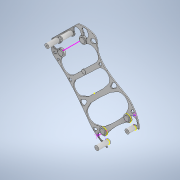
# Autodesk Inventor part: Schuh_Befestigung_alternative
Saved by Autodesk Inventor 2020.3 (Build 243373000, 373)
## iProperties
Created: 2020-03-04
Part Number: Schuh_Befestigung_alternative
Material: Generic
Document SubType Name: Modeling
Designer: Mara
Density: 1 g/cm^3
Appearance: Default
Mass: 24.396 g
Surface Area: 258.634 cm^2
Volume: 24.396 cm^3
d3: 5,563 mm
d8: 5,563 mm
d21: 60,427 mm
d22: 66,844 mm
d24: 47,207 mm
d29: 53,219 mm
d49: 6,361 mm
d51: 27,126 mm
d52: 44,927 mm
d53: 48,903 mm
d54: 29,968 mm
d55: 20,958 mm
d60: 67,034 mm
d61: 34,990 mm
d62: 27,853 mm
d63: 15,000 mm
d65: 20,850 mm
d71: 3,845 mm
d72: 5,442 mm
d73: 5,436 mm
d75: 5,541 mm
d76: 5,457 mm
d77: 3,113 mm
d78: 2,630 mm
d80: 3,207 mm
d82: 5,463 mm
d87: 1,600 mm
d88: 0,00 deg
d93: 1,000 mm
d94: 4,757 mm
d99: 1,000 mm
d100: 4,757 mm
d105: 17,100 mm
d106: 1,000 mm
d107: 0,00 deg
d108: 0,00 deg
d109: 4,757 mm
d110: 1,000 mm
d111: 11,100 mm
d112: 1,000 mm
d113: 0,00 deg
d114: 0,00 deg
d115: 2,049 mm
d117: 2,049 mm
d118: 3,300 mm
d119: 0,00 deg
d120: 2,049 mm
d121: 3,300 mm
d122: 0,00 deg
d123: 2,000 mm
d124: 0,00 deg
Author: Mara
Autodesk Inventor part; units mm, degrees
ref_plane "YZ Plane" through (0, 0, 0) normal (1, 0, 0) x (0, 1, 0)
ref_plane "XZ Plane" through (0, 0, 0) normal (0, 1, 0) x (-1, 0, 0)
ref_plane "XY Plane" through (0, 0, 0) normal (0, 0, 1) x (1, 0, 0)
sketch "Sketch1" plane through (0, 0, 0) normal (0, 0, 1) x (1, 0, 0)
  line L0 (-49.2977, 34.5359) -> (-47.8874, 33.1177) construction
  circle A0 centre (-52.4729, 29.968) radius 5.563
  circle A1 centre (-17.7815, 64.4351) radius 5.563
  circle A2 centre (14.4958, -44.9268) radius 5.563
  circle A3 centre (52.6405, -7.8239) radius 5.563
  circle A4 centre (-17.2221, 20.9576) radius 3.1804
  line L1 (-44.073, 65.9347) -> (-44.1303, 63.9354) construction
  line L2 (-59.1552, 49.3593) -> (-61.0015, 48.5894) construction
  line L3 (-42.1516, 65.9031) -> (-44.073, 65.9347) construction
  line L4 (-60.6997, 47.8234) -> (-61.0015, 48.5894) construction
  point P0 (0, 0)
  point P1 (-22.38, 61.3045)
  point P2 (-13.9364, 68.4553)
  point P3 (-12.7631, 66.8356)
  point P4 (-57.711, 28.0946)
  point P5 (-56.7093, 26.3625)
  point P6 (-49.5894, 25.2106)
  point P7 (10.1162, -41.4966)
  point P8 (9.143, -43.4122)
  point P9 (18.6755, -41.2556)
  point P10 (19.8991, -43.603)
  point P11 (47.2964, -9.3692)
  point P12 (58.0343, -9.1855)
  point P13 (55.8444, -3.2761)
  point P14 (-48.0932, 26.5378)
  point P15 (-14.6001, 59.8716)
  point P16 (48.0505, -4.6808)
  point P17 (-13.1915, 61.292)
  point P18 (49.4591, -3.2604)
  point P19 (49.4227, -12.3618)
  point P20 (19.1106, -41.8201)
  point P21 (48.0258, -10.9306)
  point P22 (17.7136, -40.3888)
  point P23 (11.2885, -49.4721)
  point P24 (9.8883, -48.0441)
  point P25 (57.2511, -4.7111)
  point P26 (55.8523, -3.2817)
  point P27 (-55.5021, 34.6339)
  point P28 (-53.6558, 35.4038)
  point P29 (-23.223, 65.5915)
  point P30 (-23.2803, 63.5921)
  point P31 (16.2732, -50.1982)
  point P32 (18.0227, -49.2289)
  point P33 (56.2951, -12.0181)
  point P34 (57.5423, -10.4544)
  point P35 (13.0651, -39.5509)
  point P36 (-16.7485, 17.8127)
  point P37 (-14.0533, 20.686)
  point P38 (47.9022, -4.9092)
  point P39 (47.1775, -6.7738)
  point P40 (-18.703, 58.9489)
  point P41 (-18.2564, 23.9652)
  point P42 (-16.7032, 58.9776)
  point P43 (-16.2565, 23.9879)
  point P44 (-47.4654, 27.5447)
  point P45 (-20.389, 20.6653)
  point P46 (-46.932, 29.4728)
  point P47 (-19.9371, 22.614)
  dimension "d3" = 5.563
  dimension "d8" = 5.563
  dimension "d21" = 60.4275
  dimension "d22" = 66.8436
  dimension "d24" = 47.2075
  dimension "d29" = 53.2188
  dimension "d49" = 6.3609
  dimension "d51" = 27.126
  dimension "d52" = 44.9268
  dimension "d53" = 48.9027
  dimension "d54" = 29.968
  dimension "d55" = 20.9576
  dimension "d60" = 67.0343
  dimension "d61" = 34.9897
  dimension "d62" = 27.8525
  dimension "d63" = 15
  dimension "d65" = 20.85
  dimension "d71" = 3.8451
  dimension "d72" = 5.4415
  dimension "d73" = 5.4358
  dimension "d75" = 5.5409
  dimension "d76" = 5.4575
  dimension "d77" = 3.1128
  dimension "d78" = 2.6305
  dimension "d80" = 3.2073
  dimension "d82" = 5.463
  dimension "d145" = 53.2132
  constraints: 10 end point, 6 point on circle, 1 centre point, 50 other
  measures "d3" distance of L0.start point (-52.473, 29.968)
  measures "d8" distance of point (-22.38, 61.305) point (-17.782, 64.435)
  measures "d21" distance of point (-52.473, 29.968) point (0, 0)
  measures "d22" distance of point (0, 0) point (-17.782, 64.435)
  measures "d24" distance of point (0, 0) point (14.496, -44.927)
  measures "d29" distance of point (0, 0) point (52.641, -7.824)
  measures "d49" diameter of A4
  measures "d51" distance of point (0, 0) A4.centre
  measures "d52" vertical distance of point (0, 0) point (14.496, -44.927)
  measures "d53" distance of point (-52.473, 29.968) point (-17.782, 64.435)
  measures "d54" vertical distance of point (0, 0) point (-52.473, 29.968)
  measures "d55" vertical distance of A4.centre point (0, 0)
  measures "d60" distance of A4.end point (47.902, -4.909)
  measures "d61" vertical distance of point (-16.703, 58.978) point (-16.256, 23.988)
  measures "d62" distance of point (-46.932, 29.473) point (-19.937, 22.614)
  measures "d63" distance of point (-53.656, 35.404) L2.start
  measures "d65" horizontal distance of point (-23.28, 63.592) L1.end
  measures "d71" horizontal distance of point (-13.936, 68.455) point (-17.782, 64.435)
  measures "d72" horizontal distance of point (-17.782, 64.435) point (-23.223, 65.591)
  measures "d73" vertical distance of point (-52.473, 29.968) point (-53.656, 35.404)
  measures "d75" horizontal distance of point (-52.473, 29.968) point (-46.932, 29.473)
  measures "d76" vertical distance of point (-17.782, 64.435) point (-16.703, 58.978)
  measures "d77" vertical distance of point (52.641, -7.824) point (57.251, -4.711)
  measures "d78" vertical distance of point (52.641, -7.824) point (57.542, -10.454)
  measures "d80" horizontal distance of point (14.496, -44.927) point (11.289, -49.472)
  measures "d82" horizontal distance of point (52.641, -7.824) point (47.178, -6.774)
  measures "d145" distance of point (52.641, -7.824) point (14.496, -44.927)
extrude "Extrusion3" add sketch "Sketch1" against normal blind 1.6
sketch "Sketch3" plane through (0, 0, 0) normal (0, 0, 1) x (1, 0, 0)
  circle A0 centre (20.7546, -56.5669) radius 2.3783
  circle A1 centre (20.7546, -56.5669) radius 3.3783
  circle A2 centre (-58.3828, 44.2123) radius 2.3783
  circle A3 centre (-58.3828, 44.2123) radius 3.3783
  circle A4 centre (52.6405, -7.8239) radius 5.563 projected
  circle A5 centre (14.4958, -44.9268) radius 5.563 projected
  point P0 (0, 0)
  point P1 (49.4227, -12.3618)
  point P2 (57.2511, -4.7111)
  point P3 (11.2885, -49.4721)
  point P4 (19.1106, -41.8201)
  dimension "d93" = 1
  dimension "d94" = 4.7566
  dimension "d99" = 1
  dimension "d100" = 4.7566
  constraints: 4 centre point, 2 coincident
  measures "d93" radial gap between concentric circles of A1 A0
  measures "d94" diameter of A0
  measures "d99" radial gap between concentric circles of A3 A2
  measures "d100" diameter of A2
extrude "Extrusion5" add sketch "Sketch3" along normal blind 17.1 and the other way blind 1 contours A1 | A3
sketch "Sketch6" plane through (0, 0, 0) normal (0, 0, 1) x (1, 0, 0)
  circle A0 centre (62.8402, -15.6905) radius 2.3785
  circle A1 centre (62.8402, -15.6905) radius 3.3785
  point P0 (0, 0)
  dimension "d109" = 4.757
  dimension "d110" = 1
  constraints: 2 centre point, 1 coincident
  measures "d109" diameter of A0
  measures "d110" radial gap between concentric circles of A1 A0
extrude "Extrusion6" add sketch "Sketch6" along normal blind 11.1 and the other way blind 1
sketch "Sketch7" plane through (-58.3828, 44.2123, 17.1) normal (0, 0, 1) x (1, 0, 0)
  circle A0 centre (0, 0) radius 3.3783
  circle A1 centre (0, 0) radius 3.3783 projected
  circle A2 centre (0, 0) radius 1.3297
  circle A3 centre (79.1375, -100.7793) radius 3.3783
  circle A4 centre (79.1375, -100.7793) radius 3.3783 projected
  circle A5 centre (79.1375, -100.7793) radius 1.3293
  point P0 (58.3828, -44.2123)
  dimension "d115" = 2.0486
  dimension "d117" = 2.049
  constraints: 4 centre point, 4 coincident, 2 concentric
  measures "d115" radial gap between concentric circles of A0 A2
  measures "d117" radial gap between concentric circles of A3 A5
extrude "Extrusion7" add sketch "Sketch7" against normal blind 3.3
sketch "Sketch8" plane through (62.8402, -15.6905, 11.1) normal (0, 0, 1) x (1, 0, 0)
  circle A0 centre (0, 0) radius 3.3785
  circle A1 centre (0, 0) radius 3.3785 projected
  circle A2 centre (0, 0) radius 1.3295
  point P0 (-62.8402, 15.6905)
  dimension "d120" = 2.049
  constraints: 2 centre point, 2 coincident, 1 concentric
  measures "d120" radial gap between concentric circles of A0 A2
extrude "Extrusion8" add sketch "Sketch8" against normal blind 3.3
sketch "Sketch9" plane through (0, 0, -1.6) normal (0, 0, -1) x (-1, 0, 0)
  circle A0 centre (58.3828, 44.2123) radius 2.3783
  circle A1 centre (58.3828, 44.2123) radius 2.3783 projected
  circle A2 centre (36.8834, 64.7402) radius 2.3783
  arc A3 (34.5051, 64.7402) -> (34.5051, 64.7402) centre (36.8834, 64.7402) ccw projected
  point P0 (0, 0)
  point P1 (56.0045, 44.2123)
  point P2 (56.0045, 44.2123)
  constraints: 2 centre point, 2 coincident, 2 concentric
extrude "Extrusion9" cut sketch "Sketch9" against normal blind 2
sketch "Sketch10" plane through (0, 0, 0) normal (0, 0, 1) x (1, 0, 0)
  circle A0 centre (52.6405, -7.8239) radius 5.563 projected
  circle A1 centre (62.8402, -15.6905) radius 3.3785 projected
  circle A2 centre (14.4958, -44.9268) radius 5.563 projected
  circle A3 centre (20.7546, -56.5669) radius 3.3783 projected
  circle A4 centre (20.7546, -56.5669) radius 3.3783 projected
  circle A5 centre (14.4958, -44.9268) radius 5.563 projected
  circle A6 centre (20.7546, -56.5669) radius 1.3293 projected
  line L0 (3.9093, -56.6581) -> (11.2885, -49.4721) projected
  circle A7 centre (62.8402, -15.6905) radius 1.3295 projected
  circle A8 centre (62.8402, -15.6905) radius 1.3295 projected
  circle A9 centre (-36.8834, 64.7402) radius 1.3293
  circle A10 centre (-36.8834, 64.7402) radius 2.3783 projected
  circle A11 centre (-58.3828, 44.2123) radius 2.3783 projected
  line L1 (-49.2977, 34.5359) -> (-22.38, 61.3045) projected
  point P0 (0, 0)
  point P1 (49.4227, -12.3618)
  point P2 (16.2829, -50.1949)
  point P3 (19.1106, -41.8201)
  point P4 (18.3621, -54.1818)
  point P5 (5.9631, -54.6581)
  point P6 (65.1179, 2.9774)
  point P7 (63.0109, 0.9182)
  point P8 (62.3382, -12.3495)
  point P9 (-57.2083, 46.2804)
  point P10 (-39.1976, 64.1914)
  point P11 (-56.04, 44.6216)
  point P12 (-37.948, 62.6134)
  constraints: 5 point on circle, 1 centre point, 1 point on line, 6 other
sketch "Sketch11" plane through (0, 0, 0) normal (0, 0, 1) x (1, 0, 0)
  circle A0 centre (-52.4729, 29.968) radius 5.563
  circle A1 centre (-52.4729, 29.968) radius 5.563 projected
  circle A2 centre (-52.4729, 29.968) radius 5.563 projected
  circle A3 centre (-52.4729, 29.968) radius 5.563 projected
  circle A4 centre (-17.7815, 64.4351) radius 5.563
  circle A5 centre (14.4958, -44.9268) radius 5.563
  circle A6 centre (52.6405, -7.8239) radius 5.563
  circle A7 centre (52.6405, -7.8239) radius 5.563 projected
  point P0 (0, 0)
  point P1 (-49.2977, 34.5359)
  point P2 (-53.6558, 35.4038)
  point P3 (-56.7093, 26.3625)
  point P4 (-49.5894, 25.2106)
  point P5 (-55.5021, 34.6339)
  point P6 (-57.711, 28.0946)
  point P7 (-13.9364, 68.4553)
  point P8 (-12.2185, 64.4351)
  point P9 (-23.223, 65.5915)
  point P10 (20.0588, -44.9268)
  point P11 (11.2885, -49.4721)
  point P12 (10.1162, -41.4966)
  point P13 (55.8523, -3.2817)
  point P14 (58.2035, -7.8239)
  point P15 (58.2035, -7.8239)
  constraints: 11 point on circle, 4 centre point, 4 concentric
extrude "Extrusion11" add sketch "Sketch11" along normal blind 0.8
sketch "Sketch12" plane through (-52.4729, 29.968, 0.8) normal (0, 0, 1) x (1, 0, 0)
  circle A0 centre (0, 0) radius 3.9985
  circle A1 centre (0, 0) radius 5.563 projected
  circle A2 centre (34.6914, 34.4671) radius 5.563 projected
  circle A3 centre (34.6914, 34.4671) radius 3.9985
  circle A4 centre (66.9687, -74.8947) radius 5.563 projected
  circle A5 centre (66.9687, -74.8947) radius 3.9985
  circle A6 centre (105.1134, -37.7919) radius 5.563 projected
  circle A7 centre (105.1134, -37.7919) radius 3.9985
  point P0 (52.4729, -29.968)
  dimension "d138" = 7.997
  dimension "d139" = 1.5645
  dimension "d140" = 7.997
  dimension "d141" = 7.997
  dimension "d142" = 7.997
  constraints: 4 centre point, 3 coincident
  measures "d138" diameter of A0
  measures "d139" radial gap between concentric circles of A0 A1
  measures "d140" diameter of A3
  measures "d141" diameter of A5
  measures "d142" diameter of A7
extrude "Extrusion12" add sketch "Sketch12" along normal blind 1 contours A0 | A3 | A5 | A7
sketch "Sketch13" plane through (-52.4729, 29.968, -1.6) normal (0, 0, -1) x (-1, 0, 0)
  arc A0 (-72.037, -95.4941) -> (-57.5443, -87.63) centre (-91.5548, -42.2379) ccw
  arc A1 (-57.5443, -87.63) -> (-44.0595, -74.0172) centre (-90.3784, -41.6193) ccw
  arc A2 (-20.5029, -42.7299) -> (-44.0595, -74.0172) centre (333.3705, -333.6762) ccw
  arc A3 (11.5166, -11.7542) -> (-20.5029, -42.7299) centre (138.9353, -175.5039) ccw
  arc A4 (16.0716, -3.8932) -> (15.4549, 11.4349) centre (-36.7536, 1.658) ccw
  arc A5 (11.5166, -11.7542) -> (16.0716, -3.8932) centre (2.1813, -1.0948) ccw
  line L0 (-25.7779, 51.9966) -> (15.4549, 11.4349)
  arc A6 (-25.7779, 51.9966) -> (-48.9728, 50.6804) centre (-34.8172, 6.2592) ccw
  arc A7 (-48.9728, 50.6804) -> (-54.7622, 45.0409) centre (-46.23, 42.0732) ccw
  arc A8 (-54.7622, 45.0409) -> (-56.0589, 39.2709) centre (-33.7926, 37.2978) ccw
  arc A9 (-56.5711, 33.7036) -> (-56.0589, 39.2709) centre (-281.8966, 57.2432) ccw
  arc A10 (-61.9243, 20.4575) -> (-56.5711, 33.7036) centre (-82.7996, 36.5985) ccw
  arc A11 (-72.0738, 10.1778) -> (-61.9243, 20.4575) centre (-99.4976, 47.4048) ccw
  arc A12 (-85.6338, 0.7644) -> (-72.0738, 10.1778) centre (-156.7554, 117.6883) ccw
  arc A13 (-103.5397, -9.3778) -> (-85.6338, 0.7644) centre (-553.714, 806.2763) ccw
  arc A14 (-103.5397, -9.3778) -> (-111.1126, -16.6996) centre (-85.4929, -35.6208) ccw
  arc A15 (-111.1126, -16.6996) -> (-120.4873, -33.6887) centre (-70.9711, -49.9311) ccw
  arc A16 (-120.4873, -33.6887) -> (-122.6827, -44.6984) centre (-77.4176, -48.0005) ccw
  line L1 (-122.6827, -44.6984) -> (-72.037, -95.4941)
  point P0 (-52.4729, -29.968)
  point P1 (-52.4749, -29.9699)
  constraints: 34 point on circle, 17 centre point, 4 end point
extrude "Extrusion13" add sketch "Sketch13" against normal blind 1.4
sketch "Sketch14" plane through (-52.4729, 29.968, -0.2) normal (0, 0, 1) x (1, 0, 0)
  arc A0 (30.7294, 38.3722) -> (19.1761, 37.6395) centre (24.7883, 40.598) ccw
  circle A1 centre (34.6914, 34.4671) radius 5.563 projected
  circle A2 centre (0, 0) radius 5.563 projected
  arc A3 (12.7593, 31.1185) -> (19.1761, 37.6395) centre (15.6189, 34.7222) ccw
  arc A4 (-8.6985, 10.4856) -> (-1.7496, 16.8027) centre (-5.8638, 14.3479) ccw
  arc A5 (-8.6985, 10.4856) -> (-14.5663, 7.4416) centre (-10.1859, 6.1752) ccw
  arc A6 (-14.5663, 7.4416) -> (-9.8157, 0) centre (-9.8062, 5.2432) ccw
  line L0 (-9.8157, 0) -> (-5.563, 0)
  arc A7 (12.7593, 31.1185) -> (-1.7496, 16.8027) centre (15.095, 14.2412) ccw
  arc A8 (38.6534, 38.3722) -> (41.5234, 48.802) centre (35.6734, 44.802) ccw
  arc A9 (41.5234, 48.802) -> (32.4139, 48.802) centre (36.9687, 47.054) ccw
  arc A10 (32.4139, 48.802) -> (34.3546, 44.168) centre (38.985, 48.8306) ccw
  arc A11 (34.6914, 40.0301) -> (34.3546, 44.168) centre (30.0196, 41.7326) ccw
  arc A12 (-10.4024, -4.3192) -> (-10.7489, -7.2712) centre (-11.1698, -5.7254) ccw
  line L1 (-10.4024, -4.3192) -> (-8.7851, -5.1021)
  line L2 (-8.7851, -5.1021) -> (-8.0664, -6.3471)
  line L3 (-8.0664, -6.3471) -> (-10.7489, -7.2712)
  arc A13 (52.4729, 37.6395) -> (49.4895, 44.168) centre (51.2863, 41.0432) ccw
  line L4 (49.4895, 44.168) -> (46.4093, 41.7326)
  line L5 (46.4093, 41.7326) -> (45.7933, 38.3722)
  line L6 (45.7933, 38.3722) -> (49.4895, 37.0246)
  line L7 (49.4895, 37.0246) -> (52.4729, 37.6395)
  arc A14 (30.7294, 38.3722) -> (38.985, 30.9299) centre (34.6914, 34.4671) ccw
  arc A15 (55.1671, 13.4743) -> (38.985, 30.9299) centre (46.4011, 21.5764) ccw
  arc A16 (1.28, -5.342) -> (19.8493, -21.2046) centre (10.9401, -12.8338) ccw
  line L8 (55.1671, 13.4743) -> (35.2508, -5.8299)
  circle A17 centre (35.2508, -9.0103) radius 3.1804 projected
  line L9 (19.8493, -21.2046) -> (32.0878, -9.3423)
  arc A18 (35.2508, -5.8299) -> (32.0878, -9.3423) centre (35.2508, -9.0103) ccw
  arc A19 (-6.871, -11.994) -> (-4.2674, -13.6642) centre (-5.4464, -12.6376) ccw
  line L10 (-4.2674, -13.6642) -> (-3.5379, -11.6631)
  line L11 (-3.5379, -11.6631) -> (-3.5379, -10.1027)
  line L12 (-3.5379, -10.1027) -> (-5.2195, -10.6821)
  line L13 (-5.2195, -10.6821) -> (-6.871, -11.994)
  arc A20 (12.2359, -29.3287) -> (15.4882, -32.0996) centre (13.862, -30.7141) ccw
  line L14 (15.4882, -32.0996) -> (16.4068, -31.287)
  line L15 (16.4068, -31.287) -> (16.5087, -29.968)
  line L16 (16.5087, -29.968) -> (15.9257, -28.4554)
  line L17 (15.9257, -28.4554) -> (13.1141, -28.5518)
  line L18 (13.1141, -28.5518) -> (12.2359, -29.3287)
  line L19 (59.4941, 15.0713) -> (60.3209, 15.9025)
  line L20 (59.2335, 12.27) -> (59.4941, 15.0713)
  line L21 (60.7094, 11.5997) -> (59.2335, 12.27)
  arc A21 (62.8971, 12.4938) -> (60.3209, 15.9025) centre (61.609, 14.1982) ccw
  line L22 (62.0321, 11.6243) -> (60.7094, 11.5997)
  line L23 (62.8971, 12.4938) -> (62.0321, 11.6243)
  arc A22 (30.7294, -54.7515) -> (37.277, -53.8855) centre (33.6979, -52.0102) ccw
  arc A23 (30.9665, -49.4464) -> (30.7294, -54.7515) centre (35.9638, -52.3276) ccw
  line L24 (37.277, -53.8855) -> (40.5855, -48.023)
  line L25 (30.9665, -49.4464) -> (38.4312, -45.8872)
  line L26 (38.4312, -45.8872) -> (40.2815, -47.1403)
  line L27 (40.2815, -47.1403) -> (40.5855, -48.023)
  arc A24 (86.5361, -0.0477) -> (81.2358, -0.3747) centre (84.2014, -5.3224) ccw
  line L28 (77.8037, -7.8987) -> (79.0881, -9.7275)
  line L29 (81.2358, -0.3747) -> (77.8037, -7.8987)
  line L30 (79.0881, -9.7275) -> (79.9758, -10.0165)
  arc A25 (85.7813, -6.609) -> (86.5361, -0.0477) centre (83.8456, -3.0622) ccw
  line L31 (85.7813, -6.609) -> (79.9758, -10.0165)
  arc A26 (73.8906, -7.0676) -> (58.0057, 6.9803) centre (65.8511, -0.1534) ccw
  arc A27 (20.6597, -29.968) -> (34.6989, -43.3595) centre (28.9526, -35.3288) ccw
  line L32 (58.0057, 6.9803) -> (21.3156, -27.7089)
  line L33 (21.3156, -27.7089) -> (20.6597, -29.968)
  line L34 (73.8906, -7.0676) -> (66.1837, -17.0703)
  line L35 (66.1837, -17.0703) -> (42.5062, -39.8702)
  line L36 (42.5062, -39.8702) -> (34.6989, -43.3595)
  arc A28 (105.6225, -25.3812) -> (86.5361, -11.0203) centre (93.8695, -21.1376) ccw
  line L37 (105.6225, -25.3812) -> (102.2106, -33.0462)
  circle A29 centre (105.1134, -37.7919) radius 5.563 projected
  line L38 (86.5361, -11.0203) -> (76.6806, -17.0499)
  line L39 (76.6806, -17.0499) -> (58.7599, -33.6007)
  line L40 (58.7599, -33.6007) -> (45.7408, -47.2708)
  line L41 (45.7408, -47.2708) -> (42.5558, -54.0083)
  arc A30 (42.5558, -54.0083) -> (56.8453, -71.9544) centre (51.9326, -61.2041) ccw
  line L42 (56.8453, -71.9544) -> (62.9636, -71.0339)
  arc A31 (38.6534, 38.3722) -> (34.6914, 40.0301) centre (34.6914, 34.4671) ccw
  arc A32 (114.4913, -25.8116) -> (111.2892, -23.4614) centre (113.0557, -24.4111) ccw
  line L43 (111.2892, -23.4614) -> (110.1208, -25.8116)
  line L44 (114.4913, -25.8116) -> (113.4337, -27.1923)
  line L45 (113.4337, -27.1923) -> (110.9367, -27.9267)
  line L46 (110.9367, -27.9267) -> (110.1208, -25.8116)
  arc A33 (50.8398, -77.9602) -> (53.4319, -81.7313) centre (52.6095, -79.5202) ccw
  line L47 (50.8398, -77.9602) -> (51.9326, -77.0845)
  line L48 (51.9326, -77.0845) -> (55.1671, -76.6058)
  line L49 (55.1671, -76.6058) -> (56.7359, -77.1778)
  arc A34 (53.4319, -81.7313) -> (56.7359, -77.1778) centre (51.0863, -76.5539) ccw
  arc A35 (119.1392, -33.3562) -> (108.6217, -33.4746) centre (113.9354, -38.3015) ccw
  circle A36 centre (115.3131, -45.6584) radius 3.3785 projected
  arc A37 (115.3131, -42.2799) -> (120.5546, -39.3326) centre (115.8018, -37.0147) ccw
  line L50 (119.1392, -33.3562) -> (120.3707, -37.5435)
  line L51 (120.3707, -37.5435) -> (120.5546, -39.3326)
  arc A38 (115.6939, -42.3015) -> (118.3936, -47.0458) centre (115.3131, -45.6584) ccw
  arc A39 (122.293, -44.0792) -> (118.3936, -47.0458) centre (123.4552, -49.6529) ccw
  line L52 (122.293, -44.0792) -> (122.3849, -44.9647)
  line L53 (122.3849, -44.9647) -> (72.2624, -95.268)
  line L54 (122.6827, -44.6984) -> (72.037, -95.4941) projected
  arc A40 (57.9036, -83.0068) -> (63.8226, -90.0936) centre (63.4958, -84.3514) ccw
  arc A41 (63.8226, -90.0936) -> (69.8492, -86.5349) centre (62.0397, -80.192) ccw
  circle A42 centre (73.2275, -86.5349) radius 3.3783 projected
  arc A43 (72.3736, -89.8035) -> (70.6812, -93.1331) centre (71.9637, -91.6901) ccw
  arc A44 (72.3736, -89.8035) -> (69.8492, -86.5349) centre (73.0546, -86.6684) ccw
  line L55 (72.2624, -95.268) -> (70.6812, -93.1331)
  circle A45 centre (66.9687, -74.8947) radius 5.563 projected
  arc A46 (63.0535, -78.8467) -> (57.9036, -83.0068) centre (63.3702, -84.5063) ccw
  circle A47 centre (66.9687, -74.8947) radius 5.563 projected
  arc A48 (66.9687, -69.3317) -> (99.5504, -37.7919) centre (-82.4899, 117.6625) ccw
  circle A49 centre (105.1134, -37.7919) radius 5.563 projected
  arc A50 (105.1134, -43.3549) -> (72.5314, -74.8308) centre (179.1023, -152.5454) ccw
  arc A51 (102.2106, -33.0462) -> (99.5504, -37.7919) centre (105.1134, -37.7919) ccw
  arc A52 (105.1134, -43.3549) -> (108.6217, -33.4746) centre (105.1134, -37.7919) ccw
  arc A53 (66.9687, -69.3317) -> (62.9636, -71.0339) centre (66.9687, -74.8947) ccw
  arc A54 (63.0535, -78.8467) -> (72.5314, -74.8308) centre (66.9687, -74.8947) ccw
  arc A55 (1.28, -5.342) -> (-5.563, 0) centre (-0.0248, 0.0405) ccw
  point P0 (52.4729, -29.968)
  point P1 (-1.7496, 16.8027)
  point P2 (1.213, -5.4291)
  point P3 (120.5546, -39.3326)
  point P4 (72.5314, -74.8308)
  point P5 (66.9687, -69.3317)
  point P6 (99.5504, -37.7919)
  constraints: 114 point on circle, 110 end point, 47 centre point, 9 concentric, 3 tangent, 2 parallel, 1 horizontal, 1 point on line, 1 vertical, 2 other
sketch "Sketch16" plane through (0, 0, -1.6) normal (0, 0, -1) x (-1, 0, 0)
  circle A0 centre (-62.8402, -15.6905) radius 2.3785 projected
  circle A1 centre (-20.7546, -56.5669) radius 2.3783 projected
  circle A2 centre (58.3828, 44.2123) radius 2.3783 projected
  circle A3 centre (36.8834, 64.7402) radius 2.3783 projected
  point P0 (0, 0)
extrude "Extrusion16" cut sketch "Sketch16" against normal up to next
extrude "Extrusion18" cut sketch "Sketch14" against normal through all contours A1 A15 L8 A17 L9 A16 A2 A55 L0 A6 A5 A4 A7 A3 A0 | A11 A10 A9 A8 A1 | A16 A55 A2 | A2 A55 A16 | A55 A2 | L1 L2 L3 A12 | L7 L6 L5 L4 A13 | L13 L12 L11 L10 A19 | L18 L17 L16 L15 L14 A20 | L19 A21 L23 L22 L21 L20 | A23 L25 L26 L27 L24 A22 | A25 L31 L30 L28 L29 A24 | L34 L35 L36 A27 L33 L32 A26 | L37 A29 A48 A45 L42 A30 L41 L40 L39 L38 A28 | A35 L50 L51 A37 A36 A39 L52 L53 L55 A43 A42 A41 A40 A46 A45 A50 A29 | L44 L45 L46 L43 A32 | L47 L48 L49 A34 A33
sketch "Sketch18" plane through (-52.4729, 29.968, -0.2) normal (0, 0, -1) x (-1, 0, 0)
  circle A0 centre (0, 0) radius 5.563
  point P0 (-52.4729, -29.968)
  constraints: 1 centre point
extrude "Extrusion19" add sketch "Sketch18" along normal blind 1.4
sketch "Sketch19" plane through (19.7895, -65.3, -1.6) normal (0.7081521, -0.7060599, 0) x (0, 0, -1)
  line L0 (-1.4, -3.7094) -> (-1.4, 1.848) projected
  line L1 (0, 71.4107) -> (0, 77.6572) projected
  line L2 (-1.4, -0.3264) -> (0, -0.3264)
  line L3 (0, -0.3264) -> (0, 71.4107)
  line L4 (0, 71.4107) -> (-1.4, 71.4107)
  line L5 (-1.4, 71.4107) -> (-1.4, -0.3264)
  point P0 (-1.6, 32.2698)
  constraints: 8 end point, 2 parallel, 1 horizontal, 1 perpendicular, 1 point on line
extrude "Extrusion20" cut sketch "Sketch19" against normal up to surface (0.0228 mm away)
fillet "Fillet7" radius 2 1 edges at (20.0585, -44.8628, -0.9)
fillet "Fillet7" radius 2 1 edges at (52.6405, -13.3869, -0.9)
fillet "Fillet7" radius 2 1 edges at (-9.9171, -24.0404, -0.9)
fillet "Fillet7" radius 2 1 edges at (-6.7321, -17.3028, -0.9)
fillet "Fillet7" radius 2 1 edges at (6.287, -3.6327, -0.9)
fillet "Fillet7" radius 2 1 edges at (24.2078, 12.918, -0.9)
fillet "Fillet7" radius 2 1 edges at (34.0632, 18.9477, -0.9)
fillet "Fillet7" radius 2 1 edges at (28.7629, 29.5932, -0.9)
fillet "Fillet7" radius 2 1 edges at (-21.5063, -19.4784, -0.9)
fillet "Fillet7" radius 2 1 edges at (-31.1573, 2.2591, -0.9)
fillet "Fillet7" radius 2 1 edges at (-31.8132, 0, -0.9)
fillet "Fillet7" radius 2 1 edges at (5.5328, 36.9483, -0.9)
fillet "Fillet7" radius 2 1 edges at (-51.2598, 24.5388, -0.9)
fillet "Fillet7" radius 2 1 edges at (-13.4879, 60.8979, -0.9)
fillet "Fillet7" radius 2 1 edges at (7.8481, 45.8705, -0.9)
fillet "Fillet7" radius 2 1 edges at (-40.237, 0.6393, -0.9)
fillet "Fillet7" radius 2 1 edges at (-67.0392, 37.4096, -0.9)
fillet "Fillet7" radius 2 1 edges at (-61.1713, 40.4536, -0.9)
fillet "Fillet7" radius 2 1 edges at (-54.2225, 46.7707, -0.9)
fillet "Fillet7" radius 2 1 edges at (-39.7136, 61.0865, -0.9)
fillet "Fillet7" radius 2 1 edges at (-33.2968, 67.6075, -0.9)
fillet "Fillet7" radius 2 1 edges at (-20.059, 78.77, -0.9)
fillet "Fillet7" radius 2 1 edges at (-18.1183, 74.136, -0.9)
fillet "Fillet7" radius 2 1 edges at (-2.9834, 74.136, -0.9)
fillet "Fillet7" radius 2 1 edges at (-6.0636, 71.7006, -0.9)
fillet "Fillet7" radius 2 2 edges at (-62.8752, 25.6488, -0.9) (-39.3588, 1.4162, -0.9)
fillet "Fillet7" radius 2 1 edges at (7.0212, 45.0392, -0.9)
fillet "Fillet7" radius 2 1 edges at (33.3084, 23.359, -0.9)
fillet "Fillet7" radius 2 1 edges at (21.4177, 22.9004, -0.9)
fillet "Fillet7" radius 2 1 edges at (13.7108, 12.8977, -0.9)
fillet "Fillet7" radius 2 1 edges at (-9.9667, -9.9023, -0.9)
fillet "Fillet7" radius 2 1 edges at (-17.774, -13.3915, -0.9)
fillet "Fillet7" radius 2 1 edges at (-15.1959, -23.9175, -0.9)
fillet "Fillet7" radius 2 1 edges at (-21.7435, 68.3402, -0.9)
fillet "Fillet7" radius 2 1 edges at (-62.2886, 29.968, -0.9)
fillet "Fillet7" radius 2 1 edges at (-36.9847, -2.1317, -0.9)
fillet "Fillet7" radius 2 1 edges at (-36.0661, -1.319, -0.9)
fillet "Fillet7" radius 2 1 edges at (-35.9642, 0, -0.9)
fillet "Fillet7" radius 2 1 edges at (-32.6236, 8.7633, -0.9)
fillet "Fillet7" radius 2 1 edges at (2.6942, 43.4423, -0.9)
fillet "Fillet7" radius 2 1 edges at (53.1496, 4.5867, -0.9)
fillet "Fillet7" radius 2 1 edges at (4.3724, -41.9864, -0.9)
fillet "Fillet7" radius 2 1 edges at (0.959, -51.7633, -0.9)
fillet "Fillet7" radius 2 1 edges at (11.3498, -60.1256, -0.9)
fillet "Fillet7" radius 2 1 edges at (68.0817, -9.3646, -0.9)
fillet "Fillet7" radius 2 1 edges at (67.8979, -7.5755, -0.9)
fillet "Fillet7" radius 2 1 edges at (62.0184, 4.1564, -0.9)
fillet "Fillet7" radius 2 1 edges at (60.9608, 2.7757, -0.9)
sketch "Sketch20" plane through (-52.4729, 29.968, -0.2) normal (0, 0, 1) x (1, 0, 0)
  circle A0 centre (15.5894, 34.7722) radius 3.3783
  circle A1 centre (15.5894, 34.7722) radius 2.3783
  circle A2 centre (15.5894, 34.7722) radius 2.3783 projected
  point P0 (52.4729, -29.968)
  dimension "d262" = 1
  constraints: 2 centre point, 2 coincident, 1 concentric
  measures "d262" radial gap between concentric circles of A0 A1
extrude "Extrusion22" add sketch "Sketch20" along normal blind 16.6
sketch "Sketch21" plane through (-36.8834, 64.7402, 16.4) normal (0, 0, 1) x (1, 0, 0)
  circle A0 centre (0, 0) radius 1.3293 projected
  circle A1 centre (0, 0) radius 3.3783
  point P0 (36.8834, -64.7402)
  dimension "d265" = 2.049
  constraints: 1 centre point, 1 coincident
  measures "d265" radial gap between concentric circles of A1 A0
extrude "Extrusion23" add sketch "Sketch21" against normal blind 3.3
equation "\"d8\" = d3"
body "Solid1"
